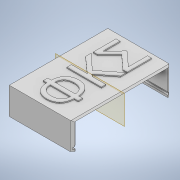
# Autodesk Inventor part: top_latch
Saved by Autodesk Inventor 2020.1 (Build 241239000, 239)
## iProperties
Created: 2019-07-05
Part Number: top_latch
Material: Generic
Document SubType Name: Modeling
Designer: jjsch
Density: 1 g/cm^3
Appearance: Default
Mass: 18.2574 g
Surface Area: 197.65 cm^2
Volume: 18.2574 cm^3
Author: jjsch
Autodesk Inventor part; units mm, degrees
ref_plane "YZ Plane" through (0, 0, 0) normal (1, 0, 0) x (0, 1, 0)
ref_plane "XZ Plane" through (0, 0, 0) normal (0, 1, 0) x (-1, 0, 0)
ref_plane "XY Plane" through (0, 0, 0) normal (0, 0, 1) x (1, 0, 0)
sketch "Sketch1" plane through (0, 0, 0) normal (0, 1, 0) x (-1, 0, 0)
  line L0 (0, 0) -> (63.837, 0)
  line L1 (63.837, 0) -> (63.837, 100)
  line L2 (63.837, 100) -> (0, 100)
  line L3 (0, 100) -> (0, 0)
  dimension "d0" = 63.837
  dimension "d1" = 100
  constraints: 8 end point, 2 parallel, 1 horizontal, 1 perpendicular
  measures "d0" distance of L2.end L1.end
  measures "d1" distance of L1.end L0.end
extrude "Extrusion1" add sketch "Sketch1" along normal blind 1.5
sketch "Sketch2" plane through (0, 0, 0) normal (0, -1, 0) x (1, 0, 0)
  line L0 (0, 100) -> (0, 0) projected
  line L1 (-63.837, 0) -> (-63.837, 100) projected
  line L2 (0, 100) -> (-63.837, 100)
  line L3 (-63.837, 100) -> (-63.837, 97)
  line L4 (-63.837, 97) -> (0, 97)
  line L5 (0, 97) -> (0, 100)
  point P0 (0, 97)
  dimension "d4" = 3
  constraints: 8 end point, 2 parallel, 1 horizontal, 1 perpendicular, 1 point on line
  measures "d4" distance of L3.end L2.end
extrude "Extrusion2" add sketch "Sketch2" along normal blind 25
sketch "Sketch3" plane through (0, 1.5, 100) normal (1, 0, 0) x (0, 0, -1)
  line L0 (3, -1.5) -> (3, -26.5) projected
  line L1 (3, -1.5) -> (100, -1.5) projected
  line L2 (3, -22.368) -> (1, -24.368)
  line L3 (3, -22.368) -> (5.8284, -22.368) construction
  line L4 (1, -24.368) -> (1, -25.368)
  line L5 (1, -25.368) -> (3, -25.368)
  line L6 (3, -22.368) -> (3, -25.368)
  dimension "d7" = 20.868
  dimension "d8" = 2.8284
  dimension "d9" = 135
  dimension "d10" = 1
  constraints: 10 end point, 2 point on line, 1 collinear, 1 equal length, 1 horizontal, 1 parallel, 1 perpendicular
  measures "d7" distance from line of L2.start L1
  measures "d8" distance of L2.start L2.end
  measures "d9" angle of L2 L3
  measures "d10" distance of L2.end L4.end
extrude "Extrusion3" cut sketch "Sketch3" against normal through all
ref_plane "Work Plane1" through (-63.837, 1.5, 50) normal (0, 0, 1) x (1, 0, 0)
mirror "Mirror1" about plane through (-63.837, 1.5, 50) normal (0, 0, 1) of "Extrusion3", "Extrusion2"
sketch "Sketch7" plane through (0, -25, 0) normal (0, -1, 0) x (1, 0, 0)
  line L0 (0, 0) -> (-63.837, 0) projected
  line L1 (0, 3) -> (0, 0) projected
  line L2 (-63.837, 3) -> (0, 3) projected
  line L3 (-63.837, 0) -> (-63.837, 3) projected
  line L4 (0, 100) -> (-63.837, 100) projected
  line L5 (-63.837, 100) -> (-63.837, 97) projected
  line L6 (-63.837, 97) -> (0, 97) projected
  line L7 (0, 97) -> (0, 100) projected
  point P0 (0, 0)
extrude "Extrusion5" add sketch "Sketch7" along normal blind 1
sketch "Sketch8" plane through (-63.837, -20.868, 3) normal (0, 0, 1) x (1, 0, 0)
  line L0 (0, -5.132) -> (0, 22.368) projected
  line L1 (0, -5.132) -> (5.419, -5.132)
  line L2 (5.419, -5.132) -> (5.419, 20.868)
  line L3 (5.419, 20.868) -> (0, 20.868)
  line L4 (0, 20.868) -> (0, -5.132)
  line L5 (0, 0) -> (63.837, 0) projected
  line L6 (0, 20.868) -> (63.837, 20.868) projected
  point P0 (0, 20.868)
  dimension "d24" = 5.419
  dimension "d26" = 0
  constraints: 8 end point, 2 parallel, 1 horizontal, 1 perpendicular
  measures "d24" distance of L3.end L2.end
  measures "d26" distance between parallel lines of L3 L6
extrude "Extrusion6" add sketch "Sketch8" along normal blind 2 and the other way blind 3
mirror "Mirror3" about plane through (-63.837, 1.5, 50) normal (0, 0, 1)
sketch "Sketch10" plane through (0, 1.5, 0) normal (0, 1, 0) x (1, 0, 0)
  line L0 (-48.837, -70) -> (-48.837, -30) construction
  line L1 (-48.837, -30) -> (-15, -30) construction
  line L2 (-15, -30) -> (-15, -70) construction
  line L3 (-15, -70) -> (-48.837, -70) construction
  line L4 (0, -97) -> (0, -3) projected
  line L5 (-63.837, 0) -> (-63.837, -100) projected
  line L6 (-63.837, -100) -> (0, -100) projected
  line L7 (0, 0) -> (-63.837, 0) projected
  spline S0 degree 2 poles (-45.9866, -75.2147) (-45.9298, -71.8963) (-43.7175, -66.3938) (-41.8739, -64.5786) knots 0 0 0 1 2 2 2
  spline S1 degree 2 poles (-41.8739, -64.5786) (-40.1438, -62.9052) (-35.2937, -61.0616) (-32.1738, -61.0616) knots 0 0 0 1 2 2 2
  spline S2 degree 2 poles (-32.1738, -61.0616) (-28.912, -61.0616) (-23.8918, -63.047) (-22.19, -64.8055) knots 0 0 0 1 2 2 2
  spline S3 degree 2 poles (-22.19, -64.8055) (-20.318, -66.7058) (-18.2475, -72.265) (-18.1908, -75.2147) knots 0 0 0 1 2 2 2
  line L8 (-18.1908, -75.2147) -> (-14.1349, -75.2147)
  line L9 (-14.1349, -75.2147) -> (-14.1349, -79.8663)
  line L10 (-14.1349, -79.8663) -> (-18.1908, -79.8663)
  spline S4 degree 2 poles (-18.1908, -79.8663) (-18.2759, -82.816) (-20.2046, -88.3468) (-22.1332, -90.3039) knots 0 0 0 1 2 2 2
  spline S5 degree 2 poles (-22.1332, -90.3039) (-23.8634, -92.0624) (-28.9404, -94.0194) (-32.1738, -94.0194) knots 0 0 0 1 2 2 2
  spline S6 degree 2 poles (-32.1738, -94.0194) (-35.237, -94.0194) (-40.0871, -92.1475) (-41.8456, -90.4457) knots 0 0 0 1 2 2 2
  spline S7 degree 2 poles (-41.8456, -90.4457) (-43.7175, -88.6305) (-45.9015, -83.1848) (-45.9866, -79.8663) knots 0 0 0 1 2 2 2
  line L11 (-45.9866, -79.8663) -> (-49.7021, -79.8663)
  line L12 (-49.7021, -79.8663) -> (-49.7021, -75.2147)
  line L13 (-49.7021, -75.2147) -> (-45.9866, -75.2147)
  spline S8 degree 2 poles (-21.7078, -75.2147) (-21.7645, -73.0875) (-23.0409, -69.7974) (-24.1187, -68.7196) knots 0 0 0 1 2 2 2
  spline S9 degree 2 poles (-24.1187, -68.7196) (-25.5368, -67.2731) (-29.5927, -65.9117) (-32.3723, -65.9117) knots 0 0 0 1 2 2 2
  spline S10 degree 2 poles (-32.3723, -65.9117) (-34.6981, -65.9117) (-38.5271, -67.2164) (-39.8602, -68.5211) knots 0 0 0 1 2 2 2
  spline S11 degree 2 poles (-39.8602, -68.5211) (-41.1365, -69.7407) (-42.3561, -72.9741) (-42.4128, -75.2147) knots 0 0 0 1 2 2 2
  line L14 (-42.4128, -75.2147) -> (-21.7078, -75.2147)
  spline S12 degree 2 poles (-42.4128, -79.8663) (-42.3845, -82.107) (-41.1081, -85.3404) (-39.8602, -86.56) knots 0 0 0 1 2 2 2
  spline S13 degree 2 poles (-39.8602, -86.56) (-38.5555, -87.8647) (-34.6414, -89.1694) (-32.3723, -89.1694) knots 0 0 0 1 2 2 2
  spline S14 degree 2 poles (-32.3723, -89.1694) (-29.5927, -89.1694) (-25.5085, -87.8079) (-24.1187, -86.3614) knots 0 0 0 1 2 2 2
  spline S15 degree 2 poles (-24.1187, -86.3614) (-23.0976, -85.2836) (-21.7362, -81.9935) (-21.7078, -79.8663) knots 0 0 0 1 2 2 2
  line L15 (-21.7078, -79.8663) -> (-42.4128, -79.8663)
  line L16 (-14.4185, -30.4579) -> (-14.4185, -36.4992)
  line L17 (-14.4185, -36.4992) -> (-30.6989, -49.2909)
  line L18 (-30.6989, -49.2909) -> (-28.4015, -51.3331)
  line L19 (-28.4015, -51.3331) -> (-14.4185, -51.3331)
  line L20 (-14.4185, -51.3331) -> (-14.4185, -55.9846)
  line L21 (-14.4185, -55.9846) -> (-49.4185, -55.9846)
  line L22 (-49.4185, -55.9846) -> (-49.4185, -51.3331)
  line L23 (-49.4185, -51.3331) -> (-33.3367, -51.3331)
  line L24 (-33.3367, -51.3331) -> (-49.4185, -36.9814)
  line L25 (-49.4185, -36.9814) -> (-49.4185, -31.3088)
  line L26 (-49.4185, -31.3088) -> (-33.7905, -45.8023)
  line L27 (-33.7905, -45.8023) -> (-14.4185, -30.4579)
  line L28 (-14.4185, -4.9595) -> (-14.4185, -29.6921)
  line L29 (-14.4185, -29.6921) -> (-18.758, -29.6921)
  line L30 (-18.758, -29.6921) -> (-32.8828, -16.8436)
  line L31 (-32.8828, -16.8436) -> (-45.2208, -29.2099)
  line L32 (-45.2208, -29.2099) -> (-49.4185, -29.2099)
  line L33 (-49.4185, -29.2099) -> (-49.4185, -6.0373)
  line L34 (-49.4185, -6.0373) -> (-45.2775, -6.0373)
  line L35 (-45.2775, -6.0373) -> (-45.2775, -23.4238)
  line L36 (-45.2775, -23.4238) -> (-33.4501, -11.3979)
  line L37 (-33.4501, -11.3979) -> (-32.8545, -11.3979)
  line L38 (-32.8545, -11.3979) -> (-18.5595, -24.4449)
  line L39 (-18.5595, -24.4449) -> (-18.5595, -4.9595)
  line L40 (-18.5595, -4.9595) -> (-14.4185, -4.9595)
  dimension "d33" = 15
  dimension "d34" = 15
  dimension "d35" = 30
  dimension "d36" = 30
  constraints: 2 other
  measures "d33" distance between parallel lines of L4 L2
  measures "d34" distance between parallel lines of L5 L0
  measures "d35" distance between parallel lines of L6 L3
  measures "d36" distance between parallel lines of L7 L1
extrude "Extrusion8" add sketch "Sketch10" along normal blind 1
chamfer "Chamfer1" distance 1.5 angle 45 1 edges at (0, 1.5, 50)
chamfer "Chamfer3" distance 2 angle 45 2 edges at (0, -13, 100) (0, -12.9999, 0)
body "Solid1"
